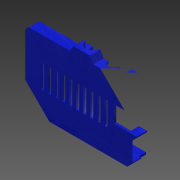
# Autodesk Inventor part: RaspiCaseUpper
Saved by Autodesk Inventor 2014 SP1 (Build 180222100, 222)
## iProperties
Created: 2014-02-10
Part Number: RaspiCaseUpper
Material: Generic
Document SubType Name: Modeling
Designer: Jack
Density: 1 g/cm^3
Appearance: Blue - Wall Paint - Glossy
Author: Jack
Autodesk Inventor part; units mm, degrees
ref_plane "YZ Plane" through (0, 0, 0) normal (1, 0, 0) x (0, 1, 0)
ref_plane "XZ Plane" through (0, 0, 0) normal (0, 1, 0) x (-1, 0, 0)
ref_plane "XY Plane" through (0, 0, 0) normal (0, 0, 1) x (1, 0, 0)
sketch "Sketch1" plane through (0, 0, 0) normal (0, 1, 0) x (-1, 0, 0)
  line L0 (0, 0) -> (90, 0)
  line L1 (90, 0) -> (90, 61)
  line L2 (90, 61) -> (0, 61)
  line L3 (0, 61) -> (0, 0)
  dimension "d0" = 90
  dimension "d1" = 61
  constraints: 8 end point, 2 perpendicular, 1 horizontal, 1 parallel
  measures "d0" distance of L0.start L0.end
  measures "d1" distance of L0.end L1.end
extrude "Extrusion1" add sketch "Sketch1" along normal blind 2
sketch "Sketch2" plane through (0, 2, 0) normal (0, 1, 0) x (1, 0, 0)
  line L0 (0, 0) -> (-90, 0) projected
  line L1 (-90, 0) -> (-90, -61) projected
  line L2 (-90, -61) -> (0, -61) projected
  line L3 (0, -61) -> (0, 0) projected
  line L4 (-88, -2) -> (-2, -2)
  line L5 (-2, -2) -> (-2, -59)
  line L6 (-2, -59) -> (-88, -59)
  line L7 (-88, -59) -> (-88, -2)
  dimension "d4" = 2
  constraints: 8 end point, 3 other
  measures "d4" distance between parallel lines of L0 L4
extrude "Extrusion2" add sketch "Sketch2" along normal blind 6.9
sketch "Sketch3" plane through (0, 0, 0) normal (0, -1, 0) x (1, 0, 0)
  line L0 (0, 61) -> (0, 0) projected
  line L1 (-90, 61) -> (0, 61) projected
  line L2 (-90, 0) -> (-90, 61) projected
  line L3 (0, 46.3) -> (5, 41.3)
  line L4 (5, 41.3) -> (5, 25.1)
  line L5 (5, 25.1) -> (0.6, 20.7)
  line L6 (0.6, 20.7) -> (0, 20.7)
  point P0 (0, 20.2)
  dimension "d7" = 45
  dimension "d8" = 14.7
  dimension "d9" = 5
  dimension "d10" = 16.2
  dimension "d18" = 0.6
  constraints: 8 end point, 3 point on line, 2 perpendicular, 1 parallel
  measures "d7" angle of L0 L3
  measures "d8" distance from line of L1 L3.start
  measures "d9" distance from line of L0 L3.end
  measures "d10" distance of L3.end L4.end
  measures "d18" distance of L5.end L6.end
extrude "Extrusion3" add sketch "Sketch3" against normal blind 8.9
sketch "Sketch4" plane through (5, 0, 41.3) normal (1, 0, 0) x (0, 0, -1)
  line L0 (16.2, 0) -> (0, 0) projected
  line L1 (0, 8.9) -> (16.2, 8.9) projected
  line L2 (0, 0) -> (0, 8.9) projected
  line L3 (15.25, 0) -> (0.95, 0)
  line L4 (0.95, 0) -> (0.95, 8.9)
  line L5 (0.95, 8.9) -> (15.25, 8.9)
  line L6 (15.25, 8.9) -> (15.25, 0)
  point P0 (41.3, 0)
  dimension "d13" = 14.3
  dimension "d14" = 0.95
  constraints: 8 end point, 2 parallel, 2 point on line, 1 horizontal, 1 perpendicular
  measures "d13" distance of L3.start L3.end
  measures "d14" distance between parallel lines of L2 L4
extrude "Extrusion4" cut sketch "Sketch4" against normal blind 19.4 contours L0 L4 L1 L6
sketch "Sketch5" plane through (-90, 0, 61) normal (0, 0, 1) x (1, 0, 0)
  line L0 (90, 0) -> (90, 8.9) projected
  line L1 (0, 8.9) -> (90, 8.9) projected
  circle A0 centre (66, 8.9) radius 4
  dimension "d19" = 8
  dimension "d20" = 24
  constraints: 1 centre point, 1 point on line
  measures "d19" diameter of A0
  measures "d20" distance from line of L0 A0.centre
extrude "Extrusion5" cut sketch "Sketch5" against normal blind 2
sketch "Sketch6" plane through (0, 0, 0) normal (0, -1, 0) x (1, 0, 0)
  line L0 (-90, 61) -> (0, 61) projected
  line L1 (5, 25.1) -> (5, 26.05) projected
  line L2 (-52, 61) -> (-49, 66)
  line L3 (-49, 66) -> (-35, 66)
  line L4 (-35, 66) -> (-32, 61)
  dimension "d23" = 5
  dimension "d24" = 3
  dimension "d25" = 3
  dimension "d26" = 32
  dimension "d27" = 14
  constraints: 6 end point, 2 point on line, 1 perpendicular
  measures "d23" distance between parallel lines of L0 L3
  measures "d24" horizontal distance of L2.end L2.start
  measures "d25" horizontal distance of L4.end L3.end
  measures "d26" distance of L0.end L4.end
  measures "d27" distance of L2.end L3.end
extrude "Extrusion6" add sketch "Sketch6" against normal blind 8.9
sketch "Sketch7" plane through (-49, 0, 66) normal (0, 0, 1) x (1, 0, 0)
  line L0 (0, 8.9) -> (14, 8.9) projected
  circle A0 centre (7, 8.9) radius 5.5
  point P0 (49, 0)
  dimension "d30" = 11
  constraints: 1 centre point, 1 midpoint
  measures "d30" diameter of A0
extrude "Extrusion7" cut sketch "Sketch7" against normal blind 13.1
sketch "Sketch8" plane through (0, 0, 0) normal (1, 0, 0) x (0, 0, -1)
  line L0 (-20.7, 8.9) -> (-20.7, 0) projected
  line L1 (-20.7, 8.9) -> (0, 8.9) projected
  line L2 (-3.8, 8.9) -> (-3.8, 1.5)
  line L3 (-3.8, 1.5) -> (-20.7, 1.5)
  dimension "d34" = 7.4
  dimension "d35" = 16.9
  constraints: 4 end point, 2 perpendicular, 2 point on line
  measures "d34" distance of L2.start L2.end
  measures "d35" distance of L2.end L3.end
extrude "Extrusion8" cut sketch "Sketch8" against normal blind 24
sketch "Sketch9" plane through (0, 2, 0) normal (0, 1, 0) x (1, 0, 0)
  line L0 (-24, -3.8) -> (-2, -3.8) projected
  line L1 (-2, -3.8) -> (-2, -2) projected
  line L2 (-88, -2) -> (-88, -59) projected
  line L3 (-2, -59) -> (-2, -40.35) projected
  line L4 (-2, -40.35) -> (-14.4, -40.35) projected
  line L5 (-2, -40.35) -> (-2, -59)
  line L6 (-2, -59) -> (-88, -59)
  line L7 (-88, -59) -> (-88, -2)
  line L8 (-88, -2) -> (-2, -2)
  line L9 (-4, -40.35) -> (-4, -57)
  line L10 (-4, -57) -> (-86, -57)
  line L11 (-86, -57) -> (-86, -4)
  line L12 (-86, -4) -> (-2, -4)
  line L13 (-2, -4) -> (-2, -2)
  line L14 (-4, -40.35) -> (-2, -40.35)
  point P0 (0, 0)
  dimension "d38" = 2
  constraints: 20 end point, 4 collinear, 2 perpendicular, 1 parallel, 3 other
  measures "d38" distance between parallel lines of L3 L9
extrude "Extrusion9" add sketch "Sketch9" along normal blind 2
sketch "Sketch10" plane through (-2, 2, 4) normal (1, 0, 0) x (0, 0, -1)
  line L0 (0.2, 0) -> (0.2, 2) projected
  line L1 (0, 2) -> (0.2, 2) projected
  line L2 (0, 0) -> (0, 2) projected
  line L3 (0, 0) -> (0.2, 0) projected
  point P0 (4, -2)
extrude "Extrusion10" cut sketch "Sketch10" against normal blind 22
sketch "Sketch11" plane through (0, 4, 0) normal (0, 1, 0) x (1, 0, 0)
  line L0 (-2, -59) -> (-39.502, -59) projected
  line L1 (-2, -40.35) -> (-2, -59) projected
  line L2 (-4, -57) -> (-86, -57) projected
  line L3 (-2, -57) -> (-14, -57)
  line L4 (-14, -57) -> (-14, -59)
  point P0 (0, 0)
  dimension "d43" = 12
  constraints: 4 end point, 3 point on line, 1 horizontal, 1 perpendicular
  measures "d43" distance of L3.start L3.end
extrude "Extrusion11" add sketch "Sketch11" along normal blind 10.9
sketch "Sketch12" plane through (0, 4, 0) normal (0, 1, 0) x (1, 0, 0)
  line L0 (-14, -57) -> (-86, -57) projected
  line L1 (-44.498, -59) -> (-88, -59) projected
  line L2 (-86, -57) -> (-86, -59)
  line L3 (-53, -57) -> (-53, -59)
  point P0 (0, 0)
  dimension "d46" = 33
  constraints: 4 end point, 3 point on line, 2 perpendicular
  measures "d46" distance between parallel lines of L3 L2
extrude "Extrusion12" cut sketch "Sketch12" against normal blind 2
sketch "Sketch13" plane through (0, 4, 0) normal (0, 1, 0) x (1, 0, 0)
  line L0 (-44.498, -59) -> (-53, -59) projected
  line L1 (-14, -57) -> (-53, -57) projected
  line L2 (-2, -3.8) -> (0, -3.8) projected
  line L3 (0, -3.8) -> (0, 0) projected
  line L4 (0, 0) -> (-90, 0) projected
  line L5 (-90, 0) -> (-90, -61) projected
  line L6 (-90, -61) -> (-52, -61) projected
  line L7 (-52, -61) -> (-49, -66) projected
  line L8 (-49, -66) -> (-47.5, -66) projected
  line L9 (-47.5, -66) -> (-47.5, -59) projected
  line L10 (-47.5, -59) -> (-88, -59) projected
  line L11 (-88, -59) -> (-88, -2) projected
  line L12 (-88, -2) -> (-2, -2) projected
  line L13 (-2, -2) -> (-2, -3.8) projected
  line L14 (-52.6, -57) -> (-52.6, -59)
  line L15 (-47.1, -57) -> (-47.1, -59)
  line L16 (-52.6, -59) -> (-47.1, -59)
  line L17 (-47.1, -57) -> (-52.6, -57)
  dimension "d49" = 5.5
  dimension "d50" = 35.4
  constraints: 8 end point, 4 point on line, 2 perpendicular, 1 collinear, 1 parallel
  measures "d49" distance between parallel lines of L14 L15
  measures "d50" distance between parallel lines of L11 L14
extrude "Extrusion13" add sketch "Sketch13" along normal blind 10.9 contours L0 L14 L1 L15
sketch "Sketch14" plane through (0, 8.9, 0) normal (0, 1, 0) x (1, 0, 0)
  line L0 (0, 0) -> (-90, 0) projected
  line L1 (-90, 0) -> (-90, -61) projected
  line L2 (-90, -61) -> (-52, -61) projected
  line L3 (-88, -59) -> (-88, -2) projected
  line L4 (-90, -5) -> (-88, -5)
  line L5 (-90, -52) -> (-88, -52)
  dimension "d53" = 9
  dimension "d54" = 5
  constraints: 4 end point, 4 point on line, 2 perpendicular
  measures "d53" distance between parallel lines of L2 L5
  measures "d54" distance between parallel lines of L0 L4
extrude "Extrusion14" add sketch "Sketch14" along normal blind 6.5
sketch "Sketch15" plane through (-90, 0, 0) normal (-1, 0, 0) x (0, 0, 1)
  line L0 (5, 15.4) -> (52, 15.4) projected
  line L1 (5, 8.9) -> (5, 15.4) projected
  line L2 (0, 0) -> (0, 8.9) projected
  line L3 (14, 15.4) -> (14, 11.4)
  line L4 (14, 11.4) -> (5, 11.4)
  dimension "d57" = 4
  dimension "d58" = 9
  constraints: 4 end point, 2 point on line, 1 parallel, 1 perpendicular
  measures "d57" distance of L3.start L3.end
  measures "d58" distance of L3.end L4.end
extrude "Extrusion15" cut sketch "Sketch15" against normal blind 2
sketch "Sketch16" plane through (0, 4, 0) normal (0, 1, 0) x (1, 0, 0)
  line L0 (-86, -4) -> (-24, -4) projected
  line L1 (-88, -2) -> (-2, -2) projected
  line L2 (-88, -59) -> (-88, -2) projected
  line L3 (-53.5, -2) -> (-53.5, -4)
  line L4 (-86, -4) -> (-88, -4)
  point P0 (0, 0)
  dimension "d61" = 34.5
  constraints: 4 end point, 3 point on line, 2 perpendicular
  measures "d61" distance between parallel lines of L2 L3
extrude "Extrusion16" add sketch "Sketch16" along normal blind 10.9
sketch "Sketch17" plane through (0, 4, 0) normal (0, 1, 0) x (1, 0, 0)
  line L0 (-24, -3.8) -> (-2, -3.8) projected
  line L1 (-2, -2) -> (-2, -3.8) projected
  line L2 (-53.5, -2) -> (-2, -2) projected
  line L3 (-17, -2) -> (-17, -3.8)
  point P0 (0, 0)
  dimension "d64" = 15
  constraints: 2 end point, 2 point on line, 1 perpendicular
  measures "d64" distance between parallel lines of L1 L3
extrude "Extrusion17" add sketch "Sketch17" along normal blind 10.9
sketch "Sketch18" plane through (0, 0, 0) normal (0, -1, 0) x (1, 0, 0)
  line L0 (0, 0) -> (-90, 0) projected
  line L1 (0, 20.7) -> (0, 0) projected
  line L2 (-20, 20.5) -> (-22.5, 20.5)
  line L3 (-22.5, 20.5) -> (-22.5, 40.5)
  line L4 (-22.5, 40.5) -> (-20, 40.5)
  line L5 (-20, 40.5) -> (-20, 20.5)
  line L6 (-26, 20.5) -> (-28.5, 20.5)
  line L7 (-28.5, 20.5) -> (-28.5, 40.5)
  line L8 (-28.5, 40.5) -> (-26, 40.5)
  line L9 (-26, 40.5) -> (-26, 20.5)
  line L10 (-32, 20.5) -> (-34.5, 20.5)
  line L11 (-34.5, 20.5) -> (-34.5, 40.5)
  line L12 (-34.5, 40.5) -> (-32, 40.5)
  line L13 (-32, 40.5) -> (-32, 20.5)
  line L14 (-38, 20.5) -> (-40.5, 20.5)
  line L15 (-40.5, 20.5) -> (-40.5, 40.5)
  line L16 (-40.5, 40.5) -> (-38, 40.5)
  line L17 (-38, 40.5) -> (-38, 20.5)
  line L18 (-44, 20.5) -> (-46.5, 20.5)
  line L19 (-46.5, 20.5) -> (-46.5, 40.5)
  line L20 (-46.5, 40.5) -> (-44, 40.5)
  line L21 (-44, 40.5) -> (-44, 20.5)
  line L22 (-50, 20.5) -> (-52.5, 20.5)
  line L23 (-52.5, 20.5) -> (-52.5, 40.5)
  line L24 (-52.5, 40.5) -> (-50, 40.5)
  line L25 (-50, 40.5) -> (-50, 20.5)
  line L26 (-56, 20.5) -> (-58.5, 20.5)
  line L27 (-58.5, 20.5) -> (-58.5, 40.5)
  line L28 (-58.5, 40.5) -> (-56, 40.5)
  line L29 (-56, 40.5) -> (-56, 20.5)
  line L30 (-62, 20.5) -> (-64.5, 20.5)
  line L31 (-64.5, 20.5) -> (-64.5, 40.5)
  line L32 (-64.5, 40.5) -> (-62, 40.5)
  line L33 (-62, 40.5) -> (-62, 20.5)
  line L34 (-68, 20.5) -> (-70.5, 20.5)
  line L35 (-70.5, 20.5) -> (-70.5, 40.5)
  line L36 (-70.5, 40.5) -> (-68, 40.5)
  line L37 (-68, 40.5) -> (-68, 20.5)
  line L38 (-74, 20.5) -> (-76.5, 20.5)
  line L39 (-76.5, 20.5) -> (-76.5, 40.5)
  line L40 (-76.5, 40.5) -> (-74, 40.5)
  line L41 (-74, 40.5) -> (-74, 20.5)
  dimension "d67" = 2.5
  dimension "d68" = 20
  dimension "d69" = 20.5
  dimension "d70" = 20
  dimension "d73" = 6
  constraints: 80 end point, 2 horizontal, 2 parallel, 1 collinear, 1 perpendicular, 71 other
  measures "d67" distance of L3.end L4.end
  measures "d68" distance of L2.end L3.end
  measures "d69" distance between parallel lines of L0 L2
  measures "d70" distance between parallel lines of L5 L1
  measures "d73" distance of L4.end L9.start
extrude "Extrusion18" cut sketch "Sketch18" against normal blind 2
sketch "Sketch20" plane through (-53.5, 8.9, 2) normal (0, 0, -1) x (-1, 0, 0)
  line L0 (34.5, 0) -> (34.5, 6) projected
  line L1 (0, 6) -> (34.5, 6) projected
  circle A0 centre (29.5, 3) radius 0.75
  point P0 (-53.5, -8.9)
  dimension "d85" = 1.5
  dimension "d86" = 3
  dimension "d87" = 5
  constraints: 1 centre point
  measures "d85" diameter of A0
  measures "d86" distance from line of L1 A0.centre
  measures "d87" distance from line of L0 A0.centre
extrude "Extrusion20" cut sketch "Sketch20" against normal blind 2
sketch "Sketch21" plane through (-14, 8.9, 59) normal (0, 0, 1) x (1, 0, 0)
  line L0 (12, 0) -> (12, 6) projected
  line L1 (0, 6) -> (12, 6) projected
  circle A0 centre (7, 3) radius 0.75
  point P0 (14, -8.9)
  dimension "d90" = 1.5
  dimension "d91" = 5
  dimension "d92" = 3
  constraints: 1 centre point
  measures "d90" diameter of A0
  measures "d91" distance from line of L0 A0.centre
  measures "d92" distance from line of L1 A0.centre
extrude "Extrusion21" cut sketch "Sketch21" against normal blind 2
chamfer "Chamfer1" distance 3 angle 45 1 edges at (-90, 4.45, 61)
chamfer "Chamfer2" distance 3 angle 45 1 edges at (-90, 4.45, 0)
chamfer "Chamfer3" distance 3 angle 45 1 edges at (0, 4.45, 0)
chamfer "Chamfer4" distance 3 angle 45 1 edges at (0, 4.45, 61)
body "Solid1"
